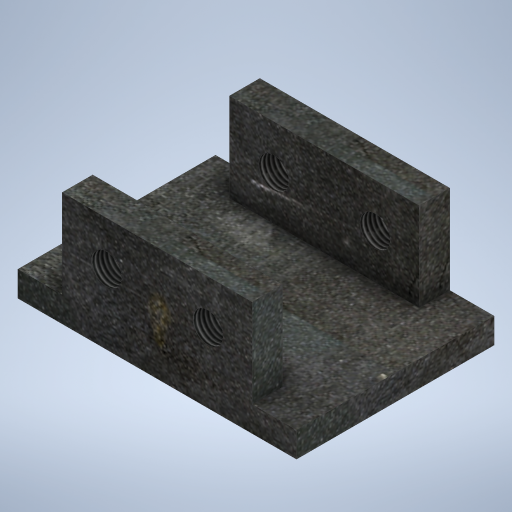
# Autodesk Inventor part: Base Macaco
Saved by Autodesk Inventor 2024 (Build 280153000, 153)
## iProperties
Created: 2024-06-01
Part Number: Base Macaco
Material: Steel ASTM A36
Document SubType Name: Modeling
Designer: Pedro
Density: 7.85 g/cm^3
Appearance: Plate
Mass: 1125.46 g
Surface Area: 340.048 cm^2
Volume: 143.371 cm^3
Author: Pedro
Autodesk Inventor part; units mm, degrees
ref_plane "YZ Plane" through (0, 0, 0) normal (1, 0, 0) x (0, 1, 0)
ref_plane "XZ Plane" through (0, 0, 0) normal (0, 1, 0) x (-1, 0, 0)
ref_plane "XY Plane" through (0, 0, 0) normal (0, 0, 1) x (1, 0, 0)
sketch "Sketch1" plane through (0, 0, 0) normal (0, 1, 0) x (-1, 0, 0)
  line L0 (55, 39) -> (55, -39)
  line L1 (55, -39) -> (-55, -39)
  line L2 (-55, -39) -> (-55, 39)
  line L3 (-55, 39) -> (55, 39)
  point P0 (0, 0)
  dimension "d0" = 78
  dimension "d1" = 110
  dimension "d2" = 55
  dimension "d3" = 39
  constraints: 8 end point, 2 parallel, 1 perpendicular, 1 vertical
  measures "d0" distance of L0.start L0.end
  measures "d1" distance of L0.end L1.end
  measures "d2" horizontal distance of L0.end point (0, 0)
  measures "d3" distance from line of L3 point (0, 0)
extrude "Extrusion1" add sketch "Sketch1" along normal blind 10
sketch "Sketch2" plane through (0, 10, 0) normal (0, 1, 0) x (1, 0, 0)
  line L0 (-37.5, -39) -> (-37.5, -27)
  line L1 (-37.5, -27) -> (37.5, -27)
  line L2 (37.5, -27) -> (37.5, -39)
  line L3 (37.5, -39) -> (-37.5, -39)
  line L4 (-55, -39) -> (55, -39) projected
  point P0 (0, 0)
  point P1 (-37.5, -33)
  dimension "d6" = 12
  dimension "d8" = 37.5
  dimension "d9" = 75
  dimension "d14" = 33
  constraints: 8 end point, 2 parallel, 1 midpoint, 1 perpendicular, 1 vertical
  measures "d6" distance of L0.start L0.end
  measures "d8" distance from line of point (0, 0) L2
  measures "d9" distance of L2.end L0.start
  measures "d14" vertical distance of point (0, 0) point (-37.5, -33)
extrude "Extrusion2" add sketch "Sketch2" along normal blind 35
sketch "Sketch3" plane through (-37.5, 45, 39) normal (0, 0, 1) x (1, 0, 0)
  circle A0 centre (17.5, -17.5) radius 6
  circle A1 centre (57.5, -17.5) radius 6
  line L0 (-17.5, -45) -> (92.5, -45) projected
  line L1 (0, 0) -> (75, 0) projected
  point P0 (37.5, -45)
  point P1 (37.5, 0)
  dimension "d16" = 12
  dimension "d17" = 12
  dimension "d18" = 27.5
  dimension "d19" = 27.5
  dimension "d20" = 40
  dimension "d21" = 20
  constraints: 2 centre point, 1 midpoint
  measures "d16" diameter of A1
  measures "d17" diameter of A0
  measures "d18" distance from line of L0 A0.centre
  measures "d19" distance from line of L0 A1.centre
  measures "d20" distance of A1.centre A0.centre
  measures "d21" horizontal distance of point (37.5, 0) A0.centre
extrude "Extrusion3" cut sketch "Sketch3" against normal blind 80
mirror "Mirror1" about plane through (0, 0, 0) normal (0, 0, 1) of "Extrusion2", "Extrusion3"
thread "Thread9" size "M12x1.75" class "6H" standard "ANSI Metric M Profile" length 350
thread "Thread13" size "M12x1.75" class "6H" standard "ANSI Metric M Profile" length 600
thread "Thread14" size "M12x1.75" class "6H" standard "ANSI Metric M Profile" length 600
thread "Thread15" size "M12x1.75" class "6H" standard "ANSI Metric M Profile" length 600
body "Solid1"
